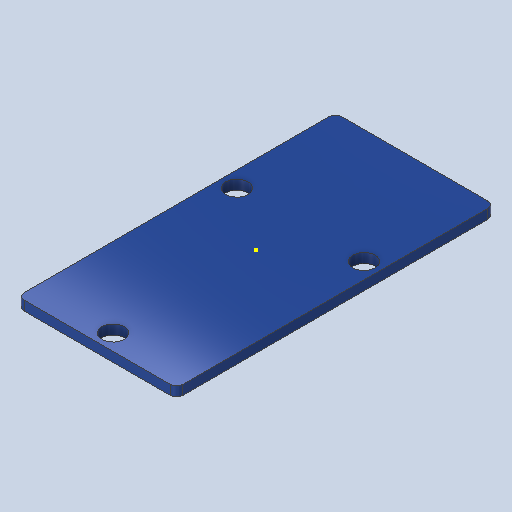
# Autodesk Inventor part: PCB
Saved by Autodesk Inventor 2023 (Build 270158000, 158)
## iProperties
Created: 2020-01-13
Part Number: PCB
Material: Générique
Document SubType Name: Modeling
Designer: thoma
Density: 1 g/cm^3
Appearance: Par défaut
Author: thoma
Autodesk Inventor part; units mm, degrees
ref_plane "YZ Plane" through (0, 0, 0) normal (1, 0, 0) x (0, 1, 0)
ref_plane "XZ Plane" through (0, 0, 0) normal (0, 1, 0) x (-1, 0, 0)
ref_plane "XY Plane" through (0, 0, 0) normal (0, 0, 1) x (1, 0, 0)
sketch "Esquisse1" plane through (0, 0, 0) normal (0, 1, 0) x (-1, 0, 0)
  line L0 (-11.5, 25) -> (11.5, 25)
  line L1 (12.5, 24) -> (12.5, -24)
  line L2 (11.5, -25) -> (-11.5, -25)
  line L3 (-12.5, -24) -> (-12.5, 24)
  line L4 (-12.5, 25) -> (12.5, -25) construction
  line L5 (12.5, 25) -> (-12.5, -25) construction
  arc A0 (12.5, 24) -> (11.5, 25) centre (11.5, 24) ccw
  arc A1 (-11.5, 25) -> (-12.5, 24) centre (-11.5, 24) ccw
  arc A2 (-12.5, -24) -> (-11.5, -25) centre (-11.5, -24) ccw
  arc A3 (11.5, -25) -> (12.5, -24) centre (11.5, -24) ccw
  line L6 (0, 25) -> (0, 22.5) construction
  circle A4 centre (0, 22.5) radius 1.75
  line L7 (9.4717, 25) -> (9.4717, -7) construction
  line L8 (12.5, -7) -> (10, -7) construction
  circle A5 centre (10, -7) radius 1.75
  circle A6 centre (-10, -7) radius 1.75
  point P0 (0, 0)
  dimension "d0" = 25
  dimension "d1" = 50
  dimension "d2" = 1
  dimension "d3" = 2.5
  dimension "d4" = 3.5
  dimension "d5" = 32
  dimension "d6" = 2.5
  dimension "d7" = 3.5
  constraints: 18 end point, 10 point on line, 8 point on circle, 8 tangent, 7 centre point, 3 equal radius, 3 midpoint, 3 parallel, 2 coincident, 2 horizontal, 1 perpendicular, 1 symmetric about line, 1 vertical, 1 other
  measures "d0" distance of L4.end L5.end
  measures "d1" distance of L5.start L4.end
  measures "d2" radius of A0
  measures "d3" distance of L6.start L6.end
  measures "d4" diameter of A4
  measures "d5" distance of L7.start L7.end
  measures "d6" distance of L8.start L8.end
  measures "d7" diameter of A5
extrude "Extrusion1" add sketch "Esquisse1" along normal blind 1.5
sketch "Sketch2" plane through (-12.5, 0, -24) normal (-1, 0, 0) x (0, 0, 1)
  point P0 (24, 0)
sketch "Sketch3" plane through (0, 1.5, 0) normal (0, 1, 0) x (1, 0, 0)
  point P0 (0, 0)
